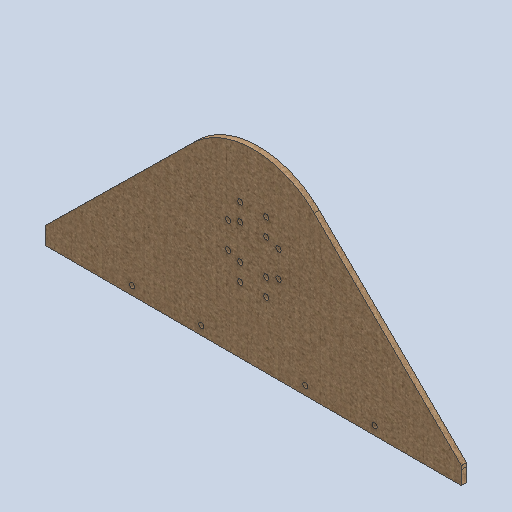
# Autodesk Inventor part: belt_liner_v1_MDF_throw_plate
Saved by Autodesk Inventor 2025.1 (Build 291241000, 241)
## iProperties
Created: 2024-12-08
Part Number: belt_liner_v1_MDF_throw_plate
Material: MDF 中密度繊維ボード
Document SubType Name: Modeling
Designer: haruy
Density: 0.8 g/cm^3
Appearance: ダンボール - 段ボール紙
Author: haruy
Autodesk Inventor part; units mm, degrees
ref_plane "YZ Plane" through (0, 0, 0) normal (1, 0, 0) x (0, 1, 0)
ref_plane "XZ Plane" through (0, 0, 0) normal (0, 1, 0) x (-1, 0, 0)
ref_plane "XY Plane" through (0, 0, 0) normal (0, 0, 1) x (1, 0, 0)
derived "belt_liner_v1_Sketch_Base.ipt"
sketch "スケッチ2" plane through (0, 0, 300) normal (0, 0, 1) x (1, 0, 0)
  circle A0 centre (0, 0) radius 120 projected
  circle A1 centre (-88.3883, -88.3883) radius 5 projected
  circle A2 centre (88.3883, -88.3883) radius 5 projected
  line L0 (0, 0) -> (0, -186.3039) projected
  line L1 (-10, 30) -> (10, 30) projected
  line L2 (10, 30) -> (10, -30) projected
  line L3 (10, -30) -> (-10, -30) projected
  line L4 (-10, -30) -> (-10, 30) projected
  line L5 (12, 2.5) -> (17, 2.5) projected
  line L6 (17, 2.5) -> (17, -2.5) projected
  line L7 (17, -2.5) -> (12, -2.5) projected
  line L8 (12, -2.5) -> (12, 2.5) projected
  circle A3 centre (-88.3883, -88.3883) radius 15 projected
  circle A4 centre (88.3883, -88.3883) radius 15 projected
  circle A5 centre (-7.5, -20) radius 1.5 projected
  circle A6 centre (-7.5, -10) radius 1.5 projected
  circle A7 centre (7.5, -10) radius 1.5 projected
  circle A8 centre (7.5, -20) radius 1.5 projected
  line L9 (0, 0) -> (10, 0) projected
  circle A9 centre (-7.5, 10) radius 1.5 projected
  circle A10 centre (-7.5, 20) radius 1.5 projected
  circle A11 centre (7.5, 10) radius 1.5 projected
  circle A12 centre (7.5, 20) radius 1.5 projected
  line L10 (12, 2.5) -> (17, 2.5) projected
  line L11 (17, 2.5) -> (17, 12.5) projected
  line L12 (17, 12.5) -> (12, 12.5) projected
  line L13 (12, 12.5) -> (12, 2.5) projected
  line L14 (12, -2.5) -> (17, -2.5) projected
  line L15 (17, -2.5) -> (17, -12.5) projected
  line L16 (17, -12.5) -> (12, -12.5) projected
  line L17 (12, -12.5) -> (12, -2.5) projected
  circle A13 centre (14.5, 7.5) radius 1.5 projected
  circle A14 centre (14.5, -7.5) radius 1.5 projected
  circle A15 centre (-14.5, 7.5) radius 1.5 projected
  circle A16 centre (-14.5, -7.5) radius 1.5 projected
  line L18 (-103.0529, -91.5429) -> (-117.3163, -25.2364) projected
  line L19 (-91.5429, -103.0529) -> (-25.2364, -117.3163) projected
  line L20 (91.5429, -103.0529) -> (25.2364, -117.3163) projected
  line L21 (103.0529, -91.5429) -> (117.3163, -25.2364) projected
  circle A17 centre (-88.3883, -88.3883) radius 1.5
  circle A18 centre (88.3883, -88.3883) radius 1.5
  circle A19 centre (0, 0) radius 130 projected
  circle A20 centre (0, 0) radius 140 projected
  line L22 (0, 0) -> (137.8731, -24.3107) projected
  line L23 (0, 0) -> (47.8828, -131.557) projected
  line L24 (0, 0) -> (121.2436, -70) projected
  circle A21 centre (46.1727, -126.8585) radius 1.5 projected
  circle A22 centre (116.9134, -67.5) radius 1.5 projected
  circle A23 centre (-46.1727, -126.8585) radius 1.5 projected
  circle A24 centre (-116.9134, -67.5) radius 1.5 projected
  line L25 (0, 0) -> (-137.8731, -24.3107) projected
  circle A25 centre (0, 0) radius 50 projected
  line L26 (-137.8731, -24.3107) -> (-25.6957, 42.8921) projected
  line L27 (137.8731, -24.3107) -> (25.6957, 42.8921) projected
  line L28 (-119.9818, -48) -> (119.9818, -48) projected
  line L29 (119.9818, -48) -> (119.9818, -58) projected
  line L30 (119.9818, -58) -> (-119.9818, -58) projected
  line L31 (-119.9818, -58) -> (-119.9818, -48) construction
  line L32 (-119.9818, -58) -> (-109.9818, -58) projected
  line L33 (-109.9818, -58) -> (-109.9818, -48) projected
  line L34 (-109.9818, -48) -> (-119.9818, -48) projected
  line L35 (-119.9818, -48) -> (-119.9818, -58) construction
  line L36 (119.9818, -58) -> (109.9818, -58) projected
  line L37 (109.9818, -58) -> (109.9818, -48) projected
  line L38 (109.9818, -48) -> (119.9818, -48) projected
  line L39 (119.9818, -48) -> (119.9818, -58) projected
  line L40 (-119.9818, -48) -> (-35.0872, 35.6214) projected
  line L41 (119.9818, -48) -> (35.0872, 35.6214) projected
  circle A26 centre (-70, -53) radius 1.5 projected
  circle A27 centre (-30, -53) radius 1.5 projected
  line L42 (-119.9818, -58) -> (-120, -58) projected
  line L43 (-120, -58) -> (-120, -48) projected
  line L44 (-120, -48) -> (-119.9818, -48) projected
  line L45 (-119.9818, -48) -> (-119.9818, -58) construction
  circle A28 centre (70, -53) radius 1.5 projected
  circle A29 centre (30, -53) radius 1.5 projected
  line L46 (120, -48) -> (119.9818, -48) projected
  line L47 (120, -58) -> (120, -48) projected
  line L48 (119.9818, -58) -> (120, -58) projected
  point P0 (25.2364, -117.3163)
  point P1 (-137.8731, -24.3107)
  point P2 (41.0424, -112.7631)
  point P3 (41.4316, -113.8325)
  point P4 (119.9818, -50.0436)
  point P5 (120, -50)
  point P6 (-35.0872, 35.6214)
  dimension "d3" = 3
  dimension "d4" = 3
  constraints: 2 centre point, 2 coincident
  measures "d3" diameter of A17
  measures "d4" diameter of A18
extrude "押し出し1" add sketch "スケッチ2" against normal blind 3 contours A25 L22 L15 L6 L11 L12 L13 L8 L2 L1 L4 L25 | L40 A25 L25 | L25 A25 L28 A0 L40 | L41 A0 L28 L24 A25 L22 | L22 A25 L41 | A0 L28 L18 L40 | L18 L28 L40 | L25 L4 L3 L0 L28 A25 | L43 L44 L28 L18 L30 A19 | A19 L30 L42 L43 | L41 L21 L28 A0 | L41 L28 L21 | A25 L24 L15 L22 | A19 L29 L46 L47 | L28 A25 L0 L30 A0 | L33 L30 L18 L28 | A0 L30 L33 | L25 L0 L3 L4 | L4 L1 L2 L9 L25 | L28 L0 A25 | L37 L30 A0 | A0 L30 L24 L28 | L28 L21 L30 L37 | L28 L29 A19 L30 L21 | L22 L7 L15 | L15 L24 A14 L17 L7 L22 | A25 L23 L2 L24 L17 L16 L15 | L24 L28 L23 A25 | L29 L30 A19 | L23 A8 L2 L3 L0 | L9 L2 L22 | L24 L2 L23 A8 | L22 L2 L24 | A25 L28 L23 L30 L0 | L0 L28 A25 | L0 L3 L2 L23 A25 L28 | L24 L30 L23 L28 | L7 L22 L8 L5 L6 | L15 L16 L17 L24 A14 | L7 L8 L22 | L23 L28 A25 | L22 L8 L17 L24 L2 | L5 L13 L12 L11
